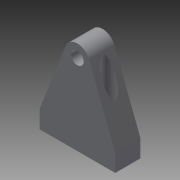
# Autodesk Inventor part: Y_axis_motor_shaft_end_support
Saved by Autodesk Inventor 2013 (Build 170138000, 138)
## iProperties
Created: 2013-09-20
Part Number: Y_axis_motor_shaft_end_support
Material: Aluminum 6061
Document SubType Name: Modeling
Designer: Ian
Density: 2.71 g/cm^3
Mass: 36.7485 g
Surface Area: 53.3535 cm^2
Volume: 13.5603 cm^3
Author: Ian
Autodesk Inventor part; units mm, degrees
ref_plane "YZ Plane" through (0, 0, 0) normal (1, 0, 0) x (0, 1, 0)
ref_plane "XZ Plane" through (0, 0, 0) normal (0, 1, 0) x (-1, 0, 0)
sketch "Sketch1" plane through (0, 0, 0) normal (0, 0, 1) x (1, 0, 0)
  line L0 (0, 0) -> (0, 40.5892) construction
  circle A0 centre (0, 40.5892) radius 3.175
  line L1 (0, 0) -> (-19.05, 0)
  arc A1 (5.9236, 42.877) -> (-5.9236, 42.877) centre (0, 40.5892) ccw
  line L2 (-19.05, 0) -> (-19.05, 8.89)
  line L3 (-19.05, 8.89) -> (-5.9236, 42.877)
  line L4 (0, 0) -> (19.05, 0)
  line L5 (19.05, 0) -> (19.05, 8.89)
  line L6 (19.05, 8.89) -> (5.9236, 42.877)
  dimension "d0" = 40.5892
  dimension "d1" = 6.35
  dimension "d3" = 19.05
  dimension "d4" = 12.7
  dimension "d7" = 8.89
  constraints: 14 end point, 3 symmetric about line, 2 centre point, 2 coincident, 2 perpendicular, 2 point on circle, 1 tangent, 1 vertical
  measures "d0" distance of L0.start L0.end
  measures "d1" diameter of A0
  measures "d3" distance of L0.start L1.end
  measures "d4" diameter of A1
  measures "d7" distance of L1.end L2.end
extrude "Extrusion1" add sketch "Sketch1" along normal blind 12.7
ref_plane "Work Plane1" through (5.9236, 42.877, 6.35) normal (0, -1, 0) x (1, 0, 0)
sketch "Sketch3" plane through (5.9236, 42.877, 6.35) normal (0, -1, 0) x (1, 0, 0)
  line L0 (3.6014, 6.1842) -> (3.6014, -6.35) construction
  circle A0 centre (3.6014, -0.0829) radius 3.175
  point P0 (-5.9236, -6.35)
  point P1 (3.6014, 6.35)
  point P2 (3.6014, 6.35)
  point P3 (3.6014, 6.35)
  dimension "d12" = 6.35
  constraints: 2 end point, 1 centre point, 1 midpoint, 1 vertical
  measures "d12" diameter of A0
extrude "Extrusion2" cut sketch "Sketch3" along normal up to surface (33.987 mm away)
mirror "Mirror1" about plane through (0, 0, 0) normal (1, 0, 0) of "Extrusion2"
body "Solid1"
